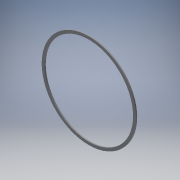
# Autodesk Inventor part: Part1
Saved by Autodesk Inventor 2017 (Build 210142000, 142)
## iProperties
Created: 2016-07-21
Part Number: Part1
Material: Generic
Document SubType Name: Modeling
Designer: Marcin
Density: 1 g/cm^3
Appearance: Default
Mass: 4963.72 g
Surface Area: 6960.51 cm^2
Volume: 4963.72 cm^3
Author: Marcin
Autodesk Inventor part; units mm, degrees
ref_plane "YZ Plane" through (0, 0, 0) normal (1, 0, 0) x (0, 1, 0)
ref_plane "XZ Plane" through (0, 0, 0) normal (0, 1, 0) x (-1, 0, 0)
ref_plane "XY Plane" through (0, 0, 0) normal (0, 0, 1) x (1, 0, 0)
sketch "Sketch1" plane through (0, 0, 0) normal (0, 1, 0) x (-1, 0, 0)
  circle A0 centre (0, 0) radius 762
  circle A1 centre (0, 0) radius 812
  dimension "d0" = 1524
  dimension "d1" = 50
  constraints: 2 centre point, 1 coincident
  measures "d0" diameter of A0
  measures "d1" radial gap between concentric circles of A0 A1
extrude "Extrusion1" add sketch "Sketch1" along normal blind 20
sketch "Sketch2" plane through (0, 20, 0) normal (0, 1, 0) x (1, 0, 0)
  circle A0 centre (788.4789, 0) radius 10
  circle A1 centre (-394.2395, 682.8428) radius 10
  circle A2 centre (-394.2395, -682.8428) radius 10
  point P0 (0, 0)
  dimension "d4" = 20
  dimension "d7" = 360
  constraints: 3 centre point, 3 other
  measures "d4" diameter of A0
extrude "Extrusion2" add sketch "Sketch2" along normal blind 20
body "Solid1"
